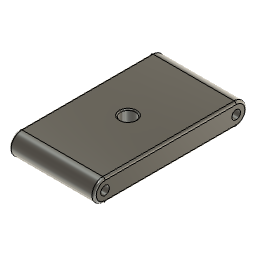
suporte_camera_fixador (Autodesk Fusion 360 design; units mm, degrees)
Autodesk Fusion 360 part; units mm, degrees
sketch "Esboço1" plane through (0, 0, 0) normal (0, 0, 1) x (1, 0, 0)
  line L0 (0, 0) -> (39, 0)
  line L1 (39, 0) -> (39, 70)
  line L2 (0, 0) -> (0, 70)
  line L3 (0, 70) -> (39, 70)
  dimension "d1" = 39
  dimension "d2" = 70
  constraint coincident L0.start L2.start
  constraint horizontal L0
  constraint vertical L1
  constraint perpendicular L0 L2
  constraint perpendicular L1 L3
  measures "d1" distance of L0.start L0.end
  measures "d2" distance of L0.end L1.end
extrude "Extrusão1" add sketch "Esboço1" along normal blind 10
sketch "Esboço3" plane through (0, 0, 0) normal (0, 0, -1) x (1, 0, 0)
  line L0 (39, 0) -> (0, 0)
  line L1 (0, 0) -> (0, -70)
  line L2 (0, -70) -> (39, -70)
  line L3 (39, -70) -> (39, 0)
  line L4 (39, 0) -> (39, -35) construction
  line L5 (39, -35) -> (0, -35) construction
  circle A0 centre (19.5, -35) radius 3.5
  dimension "d5" = 7
  constraint coincident L0.start L3.end
  constraint midpoint L3 L4.end
  constraint midpoint L1 L5.end
  constraint midpoint L5 A0.centre
  measures "d5" diameter of A0
extrude "Extrusão2" cut sketch "Esboço3" against normal blind 10 contours A0
sketch "Esboço4" plane through (0, 0, 0) normal (0, 0, -1) x (1, 0, 0)
  circle A0 centre (19.5, -35) radius 3.5
  line L0 (39, 0) -> (0, 0)
  line L1 (0, 0) -> (0, -70)
  line L2 (0, -70) -> (39, -70)
  line L3 (39, -70) -> (39, 0)
  circle A1 centre (19.5, -35) radius 6.5
  dimension "d8" = 13
  constraint concentric A0 A1
  measures "d8" diameter of A1
extrude "Extrusão3" cut sketch "Esboço4" against normal blind 3.3 contours A1
fillet "Arredondamento1" radius 5 2 edges at (19.5, 70, 10) (19.5, 70, 0)
sketch "Esboço5" plane through (0, 0, 0) normal (-1, 0, 0) x (0, -1, 0)
  arc A0 (-65, 10) -> (-65, 0) centre (-65, 5) ccw
  line L0 (-65, 0) -> (0, 0)
  line L1 (0, 0) -> (0, 10)
  line L2 (0, 10) -> (-65, 10)
  circle A1 centre (-65, 5) radius 2
  dimension "d13" = 4
  constraint concentric A0 A1
  measures "d13" diameter of A1
extrude "Extrusão4" cut sketch "Esboço5" against normal blind 40 contours A1
fillet "Arredondamento2" radius 5 2 edges at (19.5, 0, 10) (19.5, 0, 0)
sketch "Esboço6" plane through (0, 0, 0) normal (-1, 0, 0) x (0, -1, 0)
  circle A0 centre (-65, 5) radius 2
  arc A1 (-5, 0) -> (-5, 10) centre (-5, 5) ccw
  line L0 (-5, 10) -> (-65, 10)
  arc A2 (-65, 10) -> (-65, 0) centre (-65, 5) ccw
  line L1 (-65, 0) -> (-5, 0)
  circle A3 centre (-5, 5) radius 2
  dimension "d18" = 4
  constraint concentric A1 A3
  measures "d18" diameter of A3
extrude "Extrusão5" cut sketch "Esboço6" against normal blind 40 contours A3
fillet "Arredondamento3" radius 0.5 3 edges at (13.4399, 32.6495, 0) (16.2369, 36.2657, 3.3) (16.2369, 36.2657, 10)
fillet "Arredondamento4" radius 1 8 edges at (39, 70, 5) (39, 35, 10) (39, 0, 5) (39, 35, 0) (0, 35, 10) (0, 0, 5) (0, 35, 0) (0, 70, 5)
